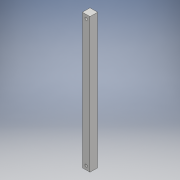
# Autodesk Inventor part: Part1
Saved by Autodesk Inventor 2018 (Build 220112000, 112)
## iProperties
Created: 2017-09-11
Part Number: Part1
Material: 一般
Document SubType Name: Modeling
Designer: Kenta
Density: 1 g/cm^3
Appearance: 既定
Author: Kenta
Autodesk Inventor part; units mm, degrees
ref_plane "YZ Plane" through (0, 0, 0) normal (1, 0, 0) x (0, 1, 0)
ref_plane "XZ Plane" through (0, 0, 0) normal (0, 1, 0) x (-1, 0, 0)
ref_plane "XY Plane" through (0, 0, 0) normal (0, 0, 1) x (1, 0, 0)
sketch "スケッチ4" plane through (0, 0, 0) normal (0, 0, 1) x (1, 0, 0)
  line L0 (-15, 15) -> (15, 15)
  line L1 (15, 15) -> (15, -15)
  line L2 (15, -15) -> (-15, -15)
  line L3 (-15, -15) -> (-15, 15)
  line L4 (-15, 15) -> (15, -15) construction
  line L5 (15, 15) -> (-15, -15) construction
  point P0 (0, 0)
  dimension "d14" = 30
  dimension "d15" = 30
  constraints: 12 end point, 2 midpoint, 2 parallel, 1 horizontal, 1 perpendicular
  measures "d14" distance of L1.end L2.end
  measures "d15" distance of L0.end L1.end
extrude "押し出し2" add sketch "スケッチ4" along normal blind 530
sketch "スケッチ5" plane through (-15, 15, 0) normal (0, 1, 0) x (1, 0, 0)
  line L0 (30, -530) -> (0, -530) projected
  line L1 (0, 0) -> (30, 0) projected
  point P0 (15, 0)
  point P1 (15, -515)
  point P2 (15, -15)
  dimension "d18" = 15
  dimension "d19" = 15
  measures "d18" distance from line of L0 point (15, -515)
  measures "d19" distance from line of point (15, -15) L1
hole "穴2" at (0, 15, 515) at (0, 15, 15) direction (0, -1, 0) diameter 10 end through all
